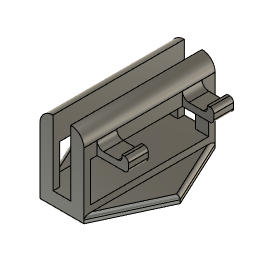
whiteboard-holder-small v5 (Autodesk Fusion 360 design; units mm, degrees)
Autodesk Fusion 360 part; units mm, degrees
note: some values were not read from the file. Set by a fixed rule: which sketch regions a step uses.
sketch "Sketch1" plane through (0, 0, 0) normal (0, 0, 1) x (1, 0, 0)
  line L0 (0, 0) -> (-13.5, 0)
  line L1 (-13.5, 0) -> (-13.5, 100)
  line L2 (-13.5, 100) -> (0, 100)
  line L3 (0, 100) -> (0, 0)
  line L4 (-13.5, 0) -> (-23.5, 0)
  line L5 (-23.5, 0) -> (-23.5, 100)
  line L6 (-23.5, 100) -> (-13.5, 100)
  line L7 (-13.5, 100) -> (-13.5, 0)
  line L8 (0, 0) -> (10, 0)
  line L9 (10, 0) -> (10, 100)
  line L10 (10, 100) -> (0, 100)
  line L11 (0, 100) -> (0, 0)
  line L12 (-23.5, 50) -> (10, 50) construction
  line L13 (33.3154, 50) -> (10, 50) construction
  line L14 (-6.75, 100) -> (-6.75, 0) construction
  line L15 (10, 100) -> (33.3154, 50)
  line L16 (33.3154, 50) -> (10, 0)
  line L17 (-23.5, 100) -> (-46.8154, 50)
  line L18 (-46.8154, 50) -> (-23.5, 0)
  dimension "d1" = 13.5
  dimension "d2" = 100
  dimension "d5" = 10
  dimension "d6" = 10
  dimension "d25" = 65
  constraint horizontal L0
  constraint vertical L1
  constraint horizontal L2
  constraint vertical L3
  constraint coincident L0.start L3.end
  constraint horizontal L4
  constraint vertical L5
  constraint horizontal L6
  constraint vertical L7
  constraint coincident L1.end L6
  constraint horizontal L8
  constraint vertical L9
  constraint horizontal L10
  constraint vertical L11
  constraint coincident L2.end L10
  constraint midpoint L5 L12.start
  constraint midpoint L9 L12.end
  constraint perpendicular L9 L13
  constraint midpoint L2 L14.start
  constraint midpoint L0 L14.end
  constraint symmetric L8.end L14 L4.end
  constraint symmetric L9.end L14 L5.end
  constraint symmetric L13.start L14 L17.end
  measures "d1" distance of L0.start L0.end
  measures "d2" distance of L0.start L2.end
  measures "d5" distance of L0.end L4.end
  measures "d6" distance of L0.start L8.end
  measures "d25" angle of L13 L15
extrude "Extrude1" add sketch "Sketch1" along normal blind 10 contours L0 L1 L2 L3 L7 L11 | L3 L8 L9 L10 L11 | L1 L4 L5 L6 L7
extrude "Extrude2" add sketch "Sketch1" along normal blind 50 from surface at 10 contours L3 L8 L9 L10 L11 | L1 L4 L5 L6 L7
fillet "Fillet1" radius 10 1 edges at (10, 50, 60)
fillet "Fillet2" radius 10 1 edges at (-23.5, 50, 60)
extrude "Extrude3" add sketch "Sketch1" along normal blind 5 contours L9 L15 L16 | L5 L17 L18
fillet "Fillet5" radius 2.5 2 edges at (21.6577, 25, 5) (21.6577, 75, 5)
fillet "Fillet6" radius 2.5 2 edges at (-35.1577, 75, 5) (-35.1577, 25, 5)
sketch "Sketch2" plane through (-23.5, 0, 0) normal (-1, 0, 0) x (0, -1, 0)
  line L0 (-94.0845, 5) -> (-5.9155, 5)
  ellipse E0 centre (-5.9155, 2.5) end of major axis (0, 2.5) minor radius 2.5 (0, 2.5) -> (-5.9155, 5) ccw
  line L1 (0, 2.5) -> (0, 50)
  line L2 (0, 50) -> (-100, 50)
  line L3 (-100, 50) -> (-100, 2.5)
  ellipse E1 centre (-94.0845, 2.5) end of major axis (-100, 2.5) minor radius 2.5 (-94.0845, 5) -> (-100, 2.5) ccw
  line L4 (-100, 2.5) -> (-100, 50)
  line L5 (-100, 50) -> (0, 50)
  line L6 (0, 2.5) -> (0, 50)
  line L7 (-94.0845, 5) -> (-5.9155, 5)
  line L8 (-95, 45) -> (-5, 45)
  line L9 (-5, 45) -> (-5, 10)
  line L10 (-5, 10) -> (-95, 10)
  line L11 (-95, 10) -> (-95, 45)
  dimension "d30" = 5
  dimension "d31" = 5
  dimension "d32" = 5
  dimension "d33" = 5
  constraint horizontal L8
  constraint vertical L9
  constraint horizontal L10
  constraint vertical L11
  measures "d30" distance of L5 L8
  measures "d31" distance of L4 L11
  measures "d32" distance of L1 L9
  measures "d33" distance of L7 L10
extrude "Extrude4" cut sketch "Sketch2" against normal blind 35 contours L8 L9 L10 L11
move_face "OffsetFaces1" offset 5 2 faces at (3.3333, 65, 45) (-20.1667, 65, 45)
sketch "Sketch3" plane through (10, 0, 0) normal (1, 0, 0) x (0, 1, 0)
  line L0 (5, 10) -> (5, 40)
  line L1 (5, 40) -> (95, 40)
  line L2 (95, 40) -> (95, 10)
  line L3 (95, 10) -> (5, 10)
  line L4 (5.9155, 5) -> (94.0845, 5)
  ellipse E0 centre (94.0845, 2.5) end of major axis (100, 2.5) minor radius 2.5 (100, 2.5) -> (94.0845, 5) ccw
  line L5 (100, 2.5) -> (100, 50)
  line L6 (100, 50) -> (0, 50)
  line L7 (0, 50) -> (0, 2.5)
  ellipse E1 centre (5.9155, 2.5) end of major axis (0, 2.5) minor radius 2.5 (5.9155, 5) -> (0, 2.5) ccw
  line L8 (0, 50) -> (100, 50)
  line L9 (0, 2.5) -> (0, 50)
  line L10 (5, 40) -> (95, 40)
  line L11 (5, 10) -> (5, 40)
  line L12 (95, 40) -> (95, 10)
  line L13 (100, 2.5) -> (100, 50)
  line L14 (95, 10) -> (5, 10)
  line L15 (50, 50) -> (50, 40) construction
  line L16 (10, 50) -> (10, 40)
  line L17 (25, 50) -> (25, 40)
  line L18 (90, 50) -> (90, 40)
  line L19 (75, 50) -> (75, 40)
  line L20 (10, 45) -> (25, 45)
  line L21 (90, 45) -> (75, 45)
  dimension "d38" = 5
  dimension "d39" = 15
  constraint midpoint L8 L15.start
  constraint midpoint L10 L15.end
  constraint coincident L8 L16.start
  constraint coincident L10 L16.end
  constraint perpendicular L10 L16
  constraint coincident L8 L17.start
  constraint coincident L10 L17.end
  constraint perpendicular L10 L17
  constraint symmetric L15 L16.start L18.start
  constraint symmetric L15 L16.end L18.end
  constraint symmetric L15 L17.start L19.start
  constraint symmetric L15 L17.end L19.end
  constraint midpoint L16 L20.start
  constraint midpoint L17 L20.end
  constraint symmetric L15 L20.start L21.start
  constraint symmetric L15 L20.end L21.end
  measures "d38" distance of L0.end L16
  measures "d39" distance of L16 L17
extrude "Extrude5" add sketch "Sketch3" along normal blind 24 contours L1 L10 L16 L17 L20 | L1 L10 L18 L19 L21
extrude "Extrude6" add sketch "Sketch3" against normal blind 5 from surface at 24 contours L6 L8 L16 L17 L20 | L6 L8 L18 L19 L21
fillet "Fillet7" radius 3 2 edges at (34, 17.5, 40) (34, 82.5, 40)
fillet "Fillet8" radius 5 2 edges at (10, 17.5, 45) (10, 82.5, 45)
fillet "Fillet9" radius 3 2 edges at (29, 17.5, 45) (29, 82.5, 45)
fillet "Fillet10" radius 3 2 edges at (34, 17.5, 50) (34, 82.5, 50)
named bodies: "small-whiteboard-holder"
